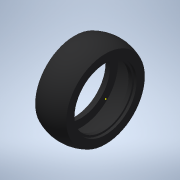
# Autodesk Inventor part: tire
Saved by Autodesk Inventor 2022.3 (Build 263350000, 350)
## iProperties
Created: 2018-01-08
Part Number: tire
Material: 고무, 검은색
Document SubType Name: Modeling
Designer: user
Density: 0.93 g/cm^3
Appearance: 고무 - 검은색
Author: user
Autodesk Inventor part; units mm, degrees
ref_plane "YZ Plane" through (0, 0, 0) normal (1, 0, 0) x (0, 1, 0)
ref_plane "XZ Plane" through (0, 0, 0) normal (0, 1, 0) x (-1, 0, 0)
ref_plane "XY Plane" through (0, 0, 0) normal (0, 0, 1) x (1, 0, 0)
sketch "스케치1" plane through (0, 0, 0) normal (0, 0, 1) x (1, 0, 0)
  line L0 (-12.5, 0) -> (12.5, 0)
  line L1 (-12.5, 31.5635) -> (-12.5, 25)
  line L2 (-12.5, 25) -> (-10.5, 25)
  line L3 (-10.5, 25) -> (-10.5, 23.5)
  line L4 (-10.5, 23.5) -> (-7.5, 23.5)
  line L5 (-7.5, 23.5) -> (-7.5, 30)
  line L6 (-7.5, 30) -> (-11.5, 30)
  line L7 (-11.5, 30) -> (-11.5, 31)
  line L8 (0, 0) -> (0, 53.0432) construction
  line L9 (12.5, 31.5635) -> (12.5, 25)
  line L10 (12.5, 25) -> (10.5, 25)
  line L11 (10.5, 25) -> (10.5, 23.5)
  line L12 (10.5, 23.5) -> (7.5, 23.5)
  line L13 (7.5, 23.5) -> (7.5, 30)
  line L14 (7.5, 30) -> (11.5, 30)
  line L15 (11.5, 30) -> (11.5, 31)
  arc A0 (11.5, 31) -> (-11.5, 31) centre (0, 3.2917) ccw
  arc A1 (12.5, 31.5635) -> (-12.5, 31.5635) centre (0, 4.2917) ccw
  dimension "d0" = 25
  dimension "d1" = 2
  dimension "d2" = 3
  dimension "d3" = 47
  dimension "d4" = 50
  dimension "d5" = 1
  dimension "d6" = 60
  dimension "d7" = 1
  dimension "d8" = 30
  dimension "d9" = 30
  dimension "d10" = 1
  constraints: 32 end point, 9 symmetric about line, 5 perpendicular, 4 point on circle, 2 centre point, 2 horizontal, 2 vertical, 1 coincident, 1 midpoint, 1 point on line, 4 other
  measures "d0" distance of L0.start L0.end
  measures "d1" distance of L1.end L2.end
  measures "d2" distance of L3.end L4.end
  measures "d3" diameter of L4 L0
  measures "d4" diameter of L2 L0
  measures "d5" distance between parallel lines of L7 L1
  measures "d6" diameter of L6 L0
  measures "d7" distance of L6.end L7.end
  measures "d8" radius of A0
  measures "d9" radius of A1
  measures "d10" distance of A1.centre A0.centre
revolve "회전1" add sketch "스케치1" angle 360 about axis through (-12.5, 0, 0) along (1, 0, 0)
sketch "Sketch2" plane through (12.5, 0, 0) normal (1, 0, 0) x (0, 0, -1)
  point P0 (0, 0)
